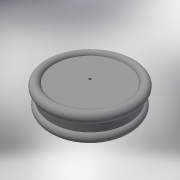
# Autodesk Inventor part: BallBalancing_Wheel
Saved by Autodesk Inventor 2016 (Build 200138000, 138)
## iProperties
Created: 2016-04-08
Part Number: BallBalancing_Wheel
Material: Generic
Document SubType Name: Modeling
Designer: Admin
Density: 1 g/cm^3
Appearance: Default
Author: Admin
Autodesk Inventor part; units mm, degrees
ref_plane "YZ Plane" through (0, 0, 0) normal (1, 0, 0) x (0, 1, 0)
ref_plane "XZ Plane" through (0, 0, 0) normal (0, 1, 0) x (-1, 0, 0)
ref_plane "XY Plane" through (0, 0, 0) normal (0, 0, 1) x (1, 0, 0)
sketch "Sketch1" plane through (0, 0, 0) normal (0, 1, 0) x (-1, 0, 0)
  line L0 (7.0899, 0) -> (-42.5397, 0) projected
  line L1 (0, -16.0296) -> (0, 16.0296) projected
  line L2 (0, -7.5) -> (-27.1459, -7.5)
  line L3 (-31.5, -3.1459) -> (-31.5, 3.1459)
  line L4 (-27.1459, 7.5) -> (0, 7.5)
  line L5 (0, 7.5) -> (0, -7.5)
  arc A0 (-31.5, -3.1459) -> (-27.1459, -7.5) centre (-30.5, -6.5) ccw
  arc A1 (-27.1459, 7.5) -> (-31.5, 3.1459) centre (-30.5, 6.5) ccw
  point P0 (0, 0)
  dimension "d1" = 7.5
  dimension "d2" = 31.5
  dimension "d4" = 1
  dimension "d5" = 1
  dimension "d6" = 7
  dimension "d7" = 7
  dimension "d8" = 1
  dimension "d9" = 1
  dimension "d10" = 15
  constraints: 8 end point, 4 point on circle, 2 centre point, 2 parallel, 1 horizontal, 1 perpendicular, 1 point on line
  measures "d1" distance between parallel lines of L0 L4
  measures "d2" distance between parallel lines of L3 L1
  measures "d4" distance from line of L2 A0.centre
  measures "d5" distance from line of L3 A0.centre
  measures "d6" diameter of A0
  measures "d7" diameter of A1
  measures "d8" distance from line of L3 A1.centre
  measures "d9" distance from line of L4 A1.centre
  measures "d10" distance between parallel lines of L2 L4
revolve "Revolution1" add sketch "Sketch1" angle 360 about axis through (0, 0, -10) along (0, 0, 1)
sketch "Sketch2" plane through (0, 0, -7.5) normal (0, 0, -1) x (-1, 0, 0)
  circle A0 centre (0, 0) radius 1
  dimension "d12" = 2
  constraints: 1 centre point, 1 coincident
  measures "d12" diameter of A0
extrude "Extrusion1" cut sketch "Sketch2" against normal through all
equation "\"d1\" = 0.5 * d10"
body "Solid1"
